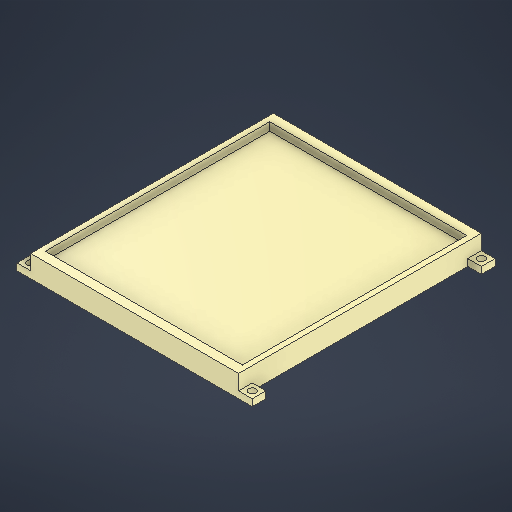
# Autodesk Inventor part: jetson_orin_nano_holder
Saved by Autodesk Inventor 2026 (Build 300175050, 175E)
## iProperties
Created: 2025-06-11
Part Number: jetson_orin_nano_holder
Material: Generic
Document SubType Name: Modeling
Designer: satom
Density: 1 g/cm^3
Appearance: Default
Author: satom
Autodesk Inventor part; units mm, degrees
ref_plane "YZ Plane" through (0, 0, 0) normal (1, 0, 0) x (0, 1, 0)
ref_plane "XZ Plane" through (0, 0, 0) normal (0, 1, 0) x (-1, 0, 0)
ref_plane "XY Plane" through (0, 0, 0) normal (0, 0, 1) x (1, 0, 0)
sketch "Sketch1" plane through (0, 0, 0) normal (0, 1, 0) x (-1, 0, 0)
  line L0 (0, 0) -> (96.52, 0)
  line L1 (96.52, 0) -> (96.52, -112.7)
  line L2 (96.52, -112.7) -> (0, -112.7)
  line L3 (0, -112.7) -> (0, 0)
  dimension "d0" = 96.52
  dimension "d1" = 112.7
  constraints: 8 end point, 2 parallel, 1 horizontal, 1 perpendicular
  measures "d0" distance of L0.start L0.end
  measures "d1" distance of L2.end L0.start
extrude "Extrusion1" add sketch "Sketch1" along normal blind 10.16
sketch "Sketch2" plane through (0, 10.16, 0) normal (0, 1, 0) x (1, 0, 0)
  line L0 (-96.52, 112.7) -> (-96.52, 0) construction
  line L1 (0, 0) -> (0, 112.7) construction
  line L2 (-96.52, 0) -> (0, 112.7) construction
  line L3 (0, 112.7) -> (-96.52, 112.7) construction
  line L4 (-96.52, 112.7) -> (0, 0) construction
  line L5 (-93.98, 4.28) -> (-2.54, 4.28)
  line L6 (-2.54, 4.28) -> (-2.54, 108.42)
  line L7 (-2.54, 108.42) -> (-93.98, 108.42)
  line L8 (-93.98, 108.42) -> (-93.98, 4.28)
  line L9 (-93.98, 4.28) -> (-2.54, 108.42) construction
  line L10 (-2.54, 4.28) -> (-93.98, 108.42) construction
  point P0 (-48.26, 56.35)
  dimension "d4" = 91.44
  dimension "d5" = 104.14
  constraints: 16 end point, 3 midpoint, 2 parallel, 1 horizontal, 1 perpendicular
  measures "d4" distance of L7.end L6.end
  measures "d5" distance of L5.end L6.end
extrude "Jetson Cavity" cut sketch "Sketch2" against normal blind 3.81
sketch "Sketch3" plane through (0, 0, 0) normal (0, -1, 0) x (1, 0, 0)
  line L0 (0, 0) -> (6.35, 0)
  line L1 (6.35, 0) -> (6.35, -6.35)
  line L2 (6.35, -6.35) -> (0, -6.35)
  line L3 (0, -6.35) -> (0, 0)
  circle A0 centre (3.175, -3.175) radius 1.7
  line L4 (6.35, -6.35) -> (0, 0) construction
  line L5 (6.35, 0) -> (0, -6.35) construction
  line L6 (0, 0) -> (0, -112.7) construction
  line L7 (0, -56.35) -> (-96.52, -56.35) construction
  line L8 (-96.52, -112.7) -> (-96.52, 0) construction
  line L9 (0, -112.7) -> (-96.52, -112.7) construction
  line L10 (-48.26, -112.7) -> (-48.26, 0) construction
  line L11 (-96.52, 0) -> (0, 0) construction
  line L12 (0, -112.7) -> (6.35, -112.7)
  line L13 (6.35, -112.7) -> (6.35, -106.35)
  line L14 (6.35, -106.35) -> (0, -106.35)
  line L15 (0, -106.35) -> (0, -112.7)
  circle A1 centre (3.175, -109.525) radius 1.7
  line L16 (6.35, -106.35) -> (0, -112.7) construction
  line L17 (6.35, -112.7) -> (0, -106.35) construction
  line L18 (-96.52, 0) -> (-102.87, 0)
  line L19 (-102.87, 0) -> (-102.87, -6.35)
  line L20 (-102.87, -6.35) -> (-96.52, -6.35)
  line L21 (-96.52, -6.35) -> (-96.52, 0)
  circle A2 centre (-99.695, -3.175) radius 1.7
  line L22 (-102.87, -6.35) -> (-96.52, 0) construction
  line L23 (-102.87, 0) -> (-96.52, -6.35) construction
  line L24 (-96.52, 0) -> (-96.52, -112.7) construction
  line L25 (-96.52, -112.7) -> (-102.87, -112.7)
  line L26 (-102.87, -112.7) -> (-102.87, -106.35)
  line L27 (-102.87, -106.35) -> (-96.52, -106.35)
  line L28 (-96.52, -106.35) -> (-96.52, -112.7)
  circle A3 centre (-99.695, -109.525) radius 1.7
  line L29 (-102.87, -106.35) -> (-96.52, -112.7) construction
  line L30 (-102.87, -112.7) -> (-96.52, -106.35) construction
  dimension "d8" = 6.35
  dimension "d9" = 6.35
  dimension "d10" = 3.4
  constraints: 54 end point, 12 symmetric about line, 5 midpoint, 4 centre point, 2 parallel, 1 horizontal, 1 perpendicular, 3 other
  measures "d8" distance of L1.end L2.end
  measures "d9" distance of L0.end L1.end
  measures "d10" diameter of A0
extrude "Screws" add sketch "Sketch3" against normal blind 3.175
sketch "Sketch4" plane through (0, 0, 0) normal (0, -1, 0) x (1, 0, 0)
  line L0 (-96.52, -112.7) -> (-96.52, 0) construction
  line L1 (0, 0) -> (-96.52, -112.7) construction
  line L2 (0, -112.7) -> (-96.52, -112.7) construction
  line L3 (-96.52, 0) -> (0, 0) construction
  line L4 (0, -112.7) -> (-96.52, 0) construction
  line L5 (-9.3482, -7.0195) -> (-87.1718, -105.6805) construction
  line L6 (-87.1718, -7.0195) -> (-9.3482, -105.6805) construction
  line L7 (-96.52, 0) -> (0, 0) construction
  line L8 (0, 0) -> (0, -112.7) construction
  line L9 (0, -112.7) -> (-96.52, -112.7) construction
  line L10 (-96.52, -112.7) -> (-96.52, 0) construction
  line L11 (-6.35, -106.35) -> (-90.17, -106.35)
  line L12 (-90.17, -106.35) -> (-90.17, -6.35)
  line L13 (-90.17, -6.35) -> (-6.35, -6.35)
  line L14 (-6.35, -6.35) -> (-6.35, -106.35)
  line L15 (-6.35, -106.35) -> (-90.17, -6.35) construction
  line L16 (-90.17, -106.35) -> (-6.35, -6.35) construction
  point P0 (-48.26, -56.35)
  point P1 (-48.26, -106.35)
  point P2 (0, -56.35)
  dimension "d14" = 6.35
  dimension "d15" = 6.35
  constraints: 28 end point, 7 midpoint, 4 parallel, 2 horizontal, 2 perpendicular
  measures "d14" distance from line of L9 point (-48.26, -106.35)
  measures "d15" distance from line of point (0, -56.35) L14
extrude "IMU Space" cut sketch "Sketch4" against normal blind 3.81
equation "\"d10\" = m3_clearance"
equation "\"m3_heat_set_insert\" = 4"
equation "\"m3_clearance\" = 3.4"
equation "\"m3_heat_set_depth\" = 7"
equation "\"robot_diameter\" = 354"
equation "\"hardboard_thickness\" = 5"
body "Solid1"
